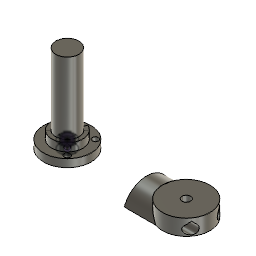
lamp_joint_first (Autodesk Fusion 360 design; units mm, degrees)
Autodesk Fusion 360 part; units mm, degrees
sketch "Sketch1" plane through (0, 0, 0) normal (0, 0, 1) x (1, 0, 0)
  circle A0 centre (0, 0) radius 7.5
  circle A1 centre (0, 0) radius 2.5
  circle A2 centre (0, 0) radius 10
  circle A3 centre (0, 0) radius 15
  line L0 (0, 0) -> (7.5, 0) construction
  line L1 (0, 0) -> (7.5, 0) construction
  line L2 (0, 0) -> (7.5, 0) construction
  line L3 (2.8701, 6.9291) -> (3.8268, 9.2388)
  line L4 (6.9291, 2.8701) -> (9.2388, 3.8268)
  dimension "d1" = 15
  dimension "d2" = 5
  dimension "d3" = 20
  dimension "d4" = 30
  constraint coincident A0.centre A1.centre
  constraint concentric A0 A2
  constraint concentric A0 A3
  constraint horizontal L0
  constraint horizontal L1
  constraint horizontal L2
  constraint coincident A2 L4.end
  measures "d1" diameter of A0
  measures "d2" diameter of A1
  measures "d3" diameter of A2
  measures "d4" diameter of A3
extrude "Extrude1" add sketch "Sketch1" along normal blind 5 contours A1 makes body 1
extrude "Extrude2" add sketch "Sketch1" along normal blind 50 contours A0 bodies 1
extrude "Extrude3" add sketch "Sketch1" along normal blind 10 from surface at 40 contours A0 A2 L3 L4 picked at (9.1313, -0.4845) bodies 1
extrude "Extrude4" add sketch "Sketch1" along normal blind 5 from surface at 45 contours A3 bodies 1
move_face "OffsetFaces1" offset -0.2 1 faces at (2.4876, -0.2489, 20) on bodies 1
sketch "Sketch2" plane through (0, 0, 50) normal (0, 0, 1) x (-1, 0, 0)
  circle A0 centre (0, 0) radius 15
  circle A1 centre (0, 0) radius 2.7
  arc A2 (-6.9291, -2.8701) -> (-2.8701, -6.9291) centre (0, 0) ccw
  line L0 (-2.8701, -6.9291) -> (-3.8268, -9.2388)
  arc A3 (-9.2388, -3.8268) -> (-3.8268, -9.2388) centre (0, 0) ccw
  line L1 (-9.2388, -3.8268) -> (-6.9291, -2.8701)
  circle A4 centre (0, 0) radius 15
  line L2 (0, 0) -> (15, 0)
  line L3 (15, 0) -> (15, -15)
  line L4 (15, 0) -> (15, 15)
  circle A5 centre (0, 0) radius 15
  line L5 (15, 0) -> (5, 0)
  line L6 (5, 0) -> (5, 14.1421)
  line L7 (5, 0) -> (5, -14.1421)
  dimension "d20" = 10
  constraint coincident A0.centre A1.centre
  constraint coincident A0 L2.end
  constraint horizontal L2
  constraint perpendicular L2 L3
  constraint perpendicular L2 L4
  constraint coincident L2.end A5
  constraint perpendicular L3 L5
  constraint coincident A5 L6.end
  constraint perpendicular L5 L6
  constraint coincident A5 L7.end
  constraint perpendicular L2 L7
  measures "d20" distance of L2.end L5.end
ref_plane "WorkPlane1" through (-15, 7.5, 50) normal (1, 0, 0) x (0, 1, 0)
extrude "Extrude5" add sketch "Sketch2" along normal blind 25 separate body contours A0 A4 L2 A5 L5 L6 | A0 A4 L2 A5 L5 L7 makes body 2
sketch "Sketch3" plane through (-5, 0, 0) normal (1, 0, 0) x (0, 1, 0)
  line L0 (14.1421, 50) -> (14.1421, 75)
  line L1 (14.1421, 75) -> (-14.1421, 75)
  line L2 (-14.1421, 75) -> (14.1421, 75)
  circle A0 centre (0, 75) radius 15
  line L3 (-14.1421, 50) -> (14.1421, 50)
  line L4 (-14.1421, 75) -> (-14.1421, 50)
  circle A1 centre (0, 75) radius 2.7
  dimension "d23" = 30
  dimension "d26" = 5.4
  constraint midpoint L1 A0.centre
  constraint concentric A0 A1
  measures "d23" diameter of A0
  measures "d26" diameter of A1
extrude "Extrude6" add sketch "Sketch3" against normal blind 10 contours L0 L1 L2 A0 L4 A1 | L0 L1 L2 A0 L4 A1 | L1 L2 A1 | L1 L2 A1 bodies 2
extrude "Extrude7" cut sketch "Sketch3" against normal blind 10 contours L1 L2 A1 | L1 L2 A1 bodies 2
move_body "Move1" bodies 1 to x (0.707107, 0.707107, 0) y (-0.707107, 0.707107, 0) z (0, 0, 1) at (0, 0, 0)
fillet "Fillet1" radius 5 1 edges at (0, 10, 50) on bodies 1
ref_plane "WorkPlane2" through (7.0711, 7.0711, 40.6713) normal (0.707107, 0.707107, 0) x (0.707107, -0.707107, 0)
sketch "Sketch4" plane through (7.0711, 7.0711, 0) normal (0.707107, 0.707107, 0) x (0.707107, -0.707107, 0)
  line L0 (-10, -40) -> (10, -40)
  line L1 (0, -40) -> (0, -42.5)
  circle A0 centre (0, -42.5) radius 1.45
  line L2 (0, -42.5) -> (1.0253, -41.4747)
  line L3 (0, -42.5) -> (1.45, -42.5) construction
  line L4 (0, -42.5) -> (-1.0253, -41.4747)
  line L5 (0, -42.5) -> (1.45, -42.5) construction
  line L6 (-1.0253, -41.4747) -> (0, -40.4494)
  line L7 (0, -40.4494) -> (1.0253, -41.4747)
  dimension "d35" = 2.5
  dimension "d36" = 2.9
  dimension "d68" = 45
  dimension "d69" = 135
  constraint midpoint L0 L1.start
  constraint perpendicular L0 L1
  constraint coincident L1.end A0.centre
  constraint horizontal L3
  constraint horizontal L5
  constraint coincident A0 L4.end
  constraint coincident L1 L6.end
  constraint tangent A0 L6
  constraint tangent A0 L7
  measures "d35" distance of L1.start L1.end
  measures "d36" diameter of A0
  measures "d68" angle of L2 L3
  measures "d69" angle of L4 L5
extrude "Extrude8" cut sketch "Sketch4" against normal blind 20 bodies 1
ref_plane "WorkPlane3" through (7.0711, -7.0711, 41.3824) normal (0.707107, -0.707107, 0) x (-0.707107, -0.707107, 0)
sketch "Sketch5" plane through (7.0711, -7.0711, 0) normal (0.707107, -0.707107, 0) x (-0.707107, -0.707107, 0)
  line L0 (-10, -40) -> (10, -40)
  line L1 (0, -40) -> (0, -42.5)
  circle A0 centre (0, -42.5) radius 1.45
  line L2 (0, -42.5) -> (1.0253, -41.4747)
  line L3 (0, -42.5) -> (1.45, -42.5) construction
  line L4 (0, -42.5) -> (-1.0253, -41.4747)
  line L5 (-1.0253, -41.4747) -> (0, -40.4494)
  line L6 (0, -40.4494) -> (1.0253, -41.4747)
  dimension "d40" = 2.5
  dimension "d41" = 2.9
  dimension "d70" = 45
  dimension "d71" = 90
  constraint midpoint L0 L1.start
  constraint perpendicular L0 L1
  constraint coincident L1.end A0.centre
  constraint horizontal L3
  constraint coincident A0 L2.end
  constraint coincident A0 L4.end
  constraint perpendicular L2 L4
  constraint coincident L1 L5.end
  measures "d40" distance of L1.start L1.end
  measures "d41" diameter of A0
  measures "d70" angle of L2 L3
  measures "d71" angle of L4 L5
extrude "Extrude9" cut sketch "Sketch5" against normal blind 20 bodies 1
move_face "OffsetFaces2" offset -0.2 1 faces at (1.9411, 7.2444, 16.6667) on bodies 1
move_face "OffsetFaces3" offset -0.2 1 faces at (-8.7595, 4.824, 42.5) on bodies 1
sketch "Sketch6" plane through (0, 0, 45) normal (0, 0, -1) x (1, 0, 0)
  arc A0 (3.7503, -9.054) -> (-3.7503, -9.054) centre (0, 0) ccw
  line L0 (3.7503, -9.054) -> (3.8268, -9.2388)
  arc A1 (-3.8268, -9.2388) -> (3.8268, -9.2388) centre (0, 0) ccw
  line L1 (-3.8268, -9.2388) -> (-3.7503, -9.054)
  circle A2 centre (0, 0) radius 15
  arc A3 (3.7503, -9.054) -> (-3.7503, -9.054) centre (0, 0) ccw
  circle A4 centre (0, 0) radius 15
  circle A5 centre (0, 0) radius 10
  line L2 (0, 0) -> (-10, 0)
  circle A6 centre (-10, 0) radius 2.5
  line L3 (0, 0) -> (-8.8388, -8.8388)
  line L4 (0, 0) -> (12.5, 0) construction
  line L5 (0, 0) -> (-8.8388, 8.8388)
  line L6 (0, 0) -> (12.5, 0) construction
  circle A7 centre (-8.8388, 8.8388) radius 1.9
  circle A8 centre (-8.8388, -8.8388) radius 1.9
  circle A9 centre (-8.8388, -8.8388) radius 1.7
  circle A10 centre (-8.8388, 8.8388) radius 1.7
  circle A11 centre (-8.8388, -8.8388) radius 3.1
  circle A12 centre (-8.8388, 8.8388) radius 3.1
  line L7 (-10, 0) -> (-17.5, 0)
  line L8 (-8.8388, 8.8388) -> (-17.5, 8.5)
  line L9 (-8.8388, -8.8388) -> (-17.5, -8.8388)
  line L10 (-8.8388, -8.8388) -> (-10.0409, -10.0409)
  line L11 (-8.8388, -8.8388) -> (-10.0409, -7.6368)
  line L12 (-10.0409, -7.6368) -> (-11.243, -8.8388)
  line L13 (-11.243, -8.8388) -> (-10.0409, -10.0409)
  line L14 (-8.8388, -8.8388) -> (-10.1823, -7.4953)
  line L15 (-10.1823, -7.4953) -> (-11.5258, -8.8388)
  line L16 (-8.8388, -8.8388) -> (-10.1823, -10.1823)
  line L17 (-10.1823, -10.1823) -> (-11.5258, -8.8388)
  line L18 (-8.8388, -8.8388) -> (-11.0309, -6.6468)
  line L19 (-8.8388, -8.8388) -> (-11.0309, -11.0309)
  line L20 (-11.0309, -11.0309) -> (-13.2229, -8.8388)
  line L21 (-13.2229, -8.8388) -> (-11.0309, -6.6468)
  line L22 (-10.1823, 10.1823) -> (-11.5258, 8.8388)
  line L23 (-10.1823, 7.4953) -> (-11.5258, 8.8388)
  line L24 (-11.243, 8.8388) -> (-10.0409, 10.0409)
  line L25 (-10.0409, 7.6368) -> (-11.243, 8.8388)
  line L26 (-8.8388, 8.8388) -> (-11.0309, 6.6468)
  line L27 (-8.8388, 8.8388) -> (-11.0309, 11.0309)
  line L28 (-13.2229, 8.8388) -> (-11.0309, 6.6468)
  line L29 (-11.0309, 11.0309) -> (-13.2229, 8.8388)
  dimension "d46" = 20
  dimension "d47" = 10
  dimension "d48" = 5
  dimension "d49" = 135
  dimension "d50" = 12.5
  dimension "d51" = 135
  dimension "d52" = 12.5
  dimension "d53" = 3.8
  dimension "d54" = 3.8
  dimension "d55" = 3.4
  dimension "d56" = 3.4
  dimension "d57" = 6.2
  dimension "d58" = 6.2
  constraint concentric A3 A4
  constraint concentric A4 A5
  constraint coincident A0.centre A1.centre
  constraint horizontal L2
  constraint coincident L2.end A6.centre
  constraint horizontal L4
  constraint horizontal L6
  constraint coincident L5.end A7.centre
  constraint coincident L3.end A8.centre
  constraint concentric A8 A9
  constraint concentric A7 A10
  constraint concentric A9 A11
  constraint concentric A7 A12
  constraint parallel L2 L7
  constraint horizontal L9
  constraint coincident A9 L10.end
  constraint parallel L3 L10
  constraint coincident A9 L11.end
  constraint perpendicular L3 L11
  constraint coincident L9 L12.end
  constraint perpendicular L11 L12
  constraint coincident A8 L14.end
  constraint perpendicular L3 L14
  constraint coincident L9 L15.end
  constraint tangent A8 L15
  constraint coincident A8 L16.end
  constraint parallel L10 L16
  constraint coincident A11 L18.end
  constraint parallel L17 L18
  constraint coincident A11 L19.end
  constraint perpendicular L18 L19
  constraint coincident L9 L20.end
  constraint tangent A11 L20
  constraint symmetric L7 L10.end L24.end
  constraint symmetric L7 L11.end L25.start
  constraint symmetric L7 L12.end L24.start
  constraint symmetric L7 L14.end L23.start
  constraint symmetric L7 L15.end L22.end
  constraint symmetric L7 L16.end L22.start
  constraint symmetric L7 L3.end L5.end
  constraint symmetric L7 L18.end L26.end
  constraint symmetric L7 L19.end L27.end
  constraint symmetric L7 L20.end L28.start
  measures "d46" diameter of A5
  measures "d47" distance of A0.centre L2.end
  measures "d48" diameter of A6
  measures "d49" angle of L3 L4
  measures "d50" distance of A0.centre L3.end
  measures "d51" angle of L5 L6
  measures "d52" distance of A0.centre L5.end
  measures "d53" diameter of A7
  measures "d54" diameter of A8
  measures "d55" diameter of A9
  measures "d56" diameter of A10
  measures "d57" diameter of A11
  measures "d58" diameter of A12
extrude "Extrude10" cut sketch "Sketch6" against normal blind 40 from surface at -5 contours L5 A10 L26 | L5 A10 L27 | A10 L8 L26 | A10 L8 L27 | A7 A10 L8 L25 | A7 L8 L25 | L3 A9 L10 L16 L19 | L3 A9 L11 L14 L18 | A7 A10 L8 L24 | A7 L8 L24 L25 | A9 L9 L10 L16 L19 | A9 L9 L11 L14 L18 | A8 A9 L9 L12 | A8 L9 L12 | A8 A9 L9 L13 | A8 L9 L13 bodies 2
extrude "Extrude11" cut sketch "Sketch6" against normal blind 5 contours L5 A7 A10 L26 | L5 A7 A10 L27 | L5 A10 L26 | L5 A10 L27 | A7 L25 L26 | L3 A8 A9 L16 L19 | L3 A8 A9 L14 L18 | A10 L8 L26 | A10 L8 L27 | A7 A10 L8 L25 | A7 L24 L27 | L3 A9 L10 L16 L19 | L3 A9 L11 L14 L18 | A8 L12 L14 L18 | A7 A10 L8 L24 | A9 L9 L10 L16 L19 | A9 L9 L11 L14 L18 | A8 A9 L9 L12 | A8 L13 L16 L19 | A8 A9 L9 L13 bodies 1
extrude "Extrude12" cut sketch "Sketch6" against normal blind 15 from surface at -30 contours A0 A3 L5 A12 | A0 A3 A5 L5 A12 | A0 A3 L5 A12 | A0 A3 A5 L5 A12 | A2 A4 A5 L5 A7 A12 L27 | A5 L5 A7 A12 L26 | A2 A4 A5 L3 A8 A11 L19 | A0 A3 A5 L3 A11 | L5 A7 A10 L26 | L5 A7 A10 L27 | A0 A3 L3 A11 | A0 A3 L3 A11 | A2 A4 A12 L27 | A5 L3 A8 A11 L18 | A0 A3 A5 L3 A11 | A2 A4 A12 L8 L28 | A12 L8 L23 L26 | A7 L8 L23 L25 | A7 L25 L26 | A2 A4 A12 L8 L22 L23 L27 | A2 A4 A12 L27 | A2 A4 A12 L8 L28 L29 | L3 A8 A9 L16 L19 | L3 A8 A9 L14 L18 | A2 A4 A11 L19 | A2 A4 A12 L8 | A2 A4 L8 L28 | A7 A10 L8 L25 | A7 L8 L25 | A7 L8 L22 L23 L24 L25 | A7 L24 L27 | A11 L9 L15 L18 | A2 A4 A11 L9 L21 | A8 L12 L14 L18 | A8 L9 L12 L15 | A2 A4 A11 L19 | A2 A4 A11 L9 L17 L19 | A2 A4 A11 L9 L20 | A7 A10 L8 L24 | A7 L8 L24 L25 | A2 A4 A11 L9 | A2 A4 L9 L21 | A8 A9 L9 L12 | A8 L9 L13 L17 | A8 L13 L16 L19 | A8 L9 L12 | A8 A9 L9 L13 | A8 L9 L13 bodies 2
move_body "Move2" bodies 2 to x (0, 0, -1) y (0, 1, 0) z (1, 0, 0) at (0, 0, 0)
ref_plane "WorkPlane4" through (0, 0, 5) normal (0, 0, -1) x (-0.707107, -0.707107, 0)
sketch "Sketch7" plane through (0, 0, 0) normal (0, 0, -1) x (1, 0, 0)
  circle A0 centre (0, 0) radius 7.3
  circle A1 centre (0, 0) radius 2.7
  dimension "d73" = 5.4
  constraint concentric A0 A1
  measures "d73" diameter of A1
sketch "Sketch8" plane through (0, 0, 5) normal (0, 0, -1) x (-1, 0, 0)
  circle A0 centre (0, 0) radius 2.7
  circle A1 centre (0, 0) radius 5
  line L0 (0, 0) -> (5, 0)
  line L1 (0, 0) -> (-5, 0)
  line L2 (0, 0) -> (0, -5)
  line L3 (0, 0) -> (0, 5)
  dimension "d76" = 5.4
  dimension "d77" = 10
  constraint coincident A0.centre A1.centre
  constraint concentric A0 A1
  constraint coincident A1 L0.end
  constraint horizontal L0
  constraint coincident A1 L1.end
  constraint parallel L0 L1
  constraint coincident A1 L2.end
  constraint perpendicular L0 L2
  constraint coincident A1 L3.end
  constraint perpendicular L0 L3
  measures "d76" diameter of A0
  measures "d77" diameter of A1
sketch "Sketch9" plane through (0, 0, 0) normal (0, 0, 1) x (1, 0, 0)
  circle A0 centre (0, 0) radius 5
  dimension "d78" = 10
  constraint coincident A0.centre origin
  measures "d78" diameter of A0
sketch "Sketch10" plane through (0, 0, 0) normal (1, 0, 0) x (0, 1, 0)
  line L0 (-5, 5) -> (5, 5)
  line L1 (0, 5) -> (-2.7, 5)
  line L2 (-2.7, 5) -> (0, 0)
  line L3 (0, 0) -> (0, 5)
  dimension "d81" = 2.7
  constraint midpoint L0 L1.start
  constraint parallel L0 L1
  constraint coincident L2.end L3.start
  measures "d81" distance of L1.start L1.end
revolve "Revolve1" add sketch "Sketch10" angle 360 about axis through (0, 0, 1.75) along (0, 0, 1) separate body makes body 3
combine "Combine1" operation cut target body 1 tool bodies 3
extrude "Extrude15" add 1 faces at (0.4428, -0.9062, 0) along direction (0, 0, -1) blind 5 on bodies 1 bodies 1
move_body "Move3" bodies 1 to x (-1, 0, 0) y (0, 1, 0) z (0, 0, -1) at (0, 0, 0)
move_body "Move4" bodies 1 to x (1, 0, 0) y (0, 1, 0) z (0, 0, 1) at (0.0004, -0.0003, 50)
move_body "Move5" bodies 2 to x (1, 0, 0) y (0, 1, 0) z (0, 0, 1) at (0, -0.0001, -5)
copy_body "Body->Comp1" bodies 1 removing the originals makes body 4 in component "Component"
copy_body "Body->Comp2" bodies 2 removing the originals makes body 5 in component "Component'"
component "Component" placed x (1, 0, 0) y (0, 1, 0) z (0, 0, 1) at (0, 0, 0)
component "Component'" placed x (1, 0, 0) y (0, 1, 0) z (0, 0, 1) at (0, 0, 0)
equation "d64 = -( 5 mm + 10 mm + 15 mm )"
